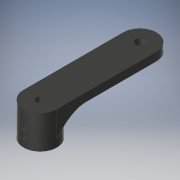
# Autodesk Inventor part: BT001_trajan20_21
Saved by Autodesk Inventor 2022.2 (Build 262287000, 287)
## iProperties
Company: HTBLA Kaindorf
RuleStatus: InUse
Created: 2022-08-07
Part Number: BT001_trajan20_21
Project: Zeichenmaschine_v2
Material: Kunststoff, undurchsichtig Schwarz
Description: gelenk 1
Document SubType Name: Modeling
Designer: trajan20
Density: 0.952 g/cm^3
Appearance: Glatt - Schwarz
Mass: 11.6591 g
Surface Area: 52.3719 cm^2
Volume: 12.2469 cm^3
AfterDocNew0: iProperties-Editor_aufrufen
Author: jan
Keywords: 2021
Autodesk Inventor part; units mm, degrees
ref_plane "YZ Plane" through (0, 0, 0) normal (1, 0, 0) x (0, 1, 0)
ref_plane "XZ Plane" through (0, 0, 0) normal (0, 1, 0) x (-1, 0, 0)
sketch "Skizze3" plane through (0, 0, 0) normal (0, 0, 1) x (1, 0, 0)
  line L0 (0, 0) -> (-60, 0) construction
  line L1 (0, 10) -> (-60, 10)
  line L2 (-60, -10) -> (0, -10)
  arc A0 (0, -10) -> (0, 10) centre (0, 0) ccw
  arc A1 (-60, 10) -> (-60, -10) centre (-60, 0) ccw
  circle A2 centre (0, 0) radius 2.5
  circle A3 centre (-60, 0) radius 2.75
  point P0 (-30, 0)
  point P1 (-40, 0)
  dimension "d4" = 60
  dimension "d5" = 20
  dimension "d6" = 5.5
  dimension "d7" = 5
  dimension "d8" = 40
  constraints: 8 end point, 4 centre point, 4 point on circle, 4 tangent, 2 coincident, 1 horizontal, 1 midpoint, 1 parallel, 1 point on line
  measures "d4" distance of L0.end L0.start
  measures "d5" distance between parallel lines of L2 L1
  measures "d6" diameter of A3
  measures "d7" diameter of A2
  measures "d8" distance of L0.start point (-40, 0)
extrude "Extrusion3" add sketch "Skizze3" along normal blind 5
sketch "Skizze5" plane through (0, 0, 0) normal (0, 0, -1) x (-1, 0, 0)
  circle A0 centre (0, 0) radius 2.5 projected
  circle A1 centre (0, 0) radius 10
  line L0 (0, 10) -> (60, 10) projected
  constraints: 1 coincident, 1 horizontal, 1 vertical alignment, 1 other
extrude "Extrusion4" add sketch "Skizze5" along normal blind 15
fillet "Rundung1" radius 10 2 edges at (-7.0711, 7.0711, 0) (-7.0711, -7.0711, 0)
ref_plane "Arbeitsebene1" through (10, 0, 5) normal (1, 0, 0) x (0, 1, 0)
sketch "Skizze7" plane through (10, 0, 5) normal (1, 0, 0) x (0, 1, 0)
  line L0 (-2.5, 0) -> (-2.5, -20) projected
  line L1 (-2.5, 0) -> (-2.5, -20) projected
  line L2 (2.5, 0) -> (2.5, -20) projected
  line L3 (2.5, 0) -> (2.5, -20) projected
  line L4 (0, -6.4797) -> (0, -2.8398) construction
  line L5 (-10, -20) -> (10, -20) projected
  line L6 (-10, -5) -> (10, -5) projected
  point P0 (0, -5)
  point P1 (0, -10)
  point P2 (0, -15)
  dimension "d30" = 5
  dimension "d31" = 5
  constraints: 3 point on line, 2 end point, 1 vertical
  measures "d30" distance from line of L5 point (0, -15)
  measures "d31" distance from line of L6 point (0, -10)
hole "Bohrung3" at (10, 0, -5) at (10, 0, -10) direction (-1, 0, 0) diameter 2.013 end up to surface thread size "M2.5x0.45" class "6H" standard "ISO Metric profile"
equation "\"d31\" = d30"
